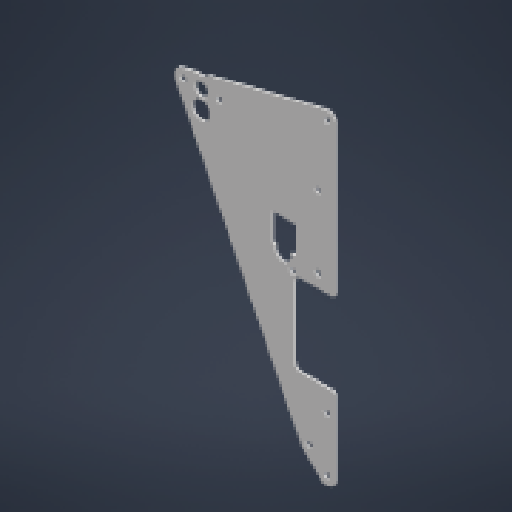
# Autodesk Inventor part: outer-tower-support-proto
Saved by Autodesk Inventor 2023 (Build 270158000, 158)
## iProperties
Created: 2023-03-21
Part Number: outer-tower-support-proto
Material: Generic
Document SubType Name: Modeling
Designer: Liam
Density: 1 g/cm^3
Appearance: Default
Author: Liam
Autodesk Inventor part; units mm, degrees
ref_plane "YZ Plane" through (0, 0, 0) normal (1, 0, 0) x (0, 1, 0)
ref_plane "XZ Plane" through (0, 0, 0) normal (0, 1, 0) x (-1, 0, 0)
ref_plane "XY Plane" through (0, 0, 0) normal (0, 0, 1) x (1, 0, 0)
sketch "Sketch1" plane through (0, 0, 0) normal (0, 0, 1) x (1, 0, 0)
  circle A0 centre (-71.4375, -30.1625) radius 6.35
  line L0 (12.9724, -214.0401) -> (0.2724, -201.3401)
  line L1 (-0.9271, -199.6696) -> (-89.8271, -20.2821)
  line L2 (23.8157, 7.5349) -> (23.8157, -44.8526)
  arc A1 (12.9724, -214.0401) -> (23.8125, -209.55) centre (17.4625, -209.55) ccw
  arc A2 (-0.9271, -199.6696) -> (0.2724, -201.3401) centre (4.7625, -196.85) ccw
  arc A3 (-85.6776, -11.3021) -> (-89.8271, -20.2821) centre (-84.1375, -17.4625) ccw
  arc A4 (23.8157, 7.5349) -> (15.9224, 14.0979) centre (17.4787, 7.9416) ccw
  circle A5 centre (-71.4375, -17.4625) radius 2.1844
  line L3 (-85.6776, -11.3021) -> (-75.211, -8.6854)
  line L4 (15.9224, 14.0979) -> (-66.2619, -6.4482)
  arc A6 (-73.1895, -8.8477) -> (-67.9692, -7.5426) centre (-71.4375, -4.7625) ccw
  arc A7 (-66.2619, -6.4482) -> (-67.9692, -7.5426) centre (-65.4918, -9.5284) ccw
  arc A8 (-73.1895, -8.8477) -> (-75.211, -8.6854) centre (-74.4409, -11.7656) ccw
  circle A9 centre (-71.4375, -17.4625) radius 4.445
  circle A10 centre (11.1125, -88.9) radius 2.2098
  line L5 (23.8125, -159.2779) -> (23.8125, -209.55)
  line L6 (23.8157, -44.8526) -> (23.8157, -94.965)
  circle A11 centre (17.4787, 7.9416) radius 2.1082
  circle A12 centre (-84.1375, -17.4625) radius 2.1082
  circle A13 centre (-58.7375, -17.4625) radius 2.1844 projected
  circle A14 centre (11.1125, -38.1) radius 2.1844 projected
  circle A15 centre (17.4625, -209.55) radius 2.1082
  circle A16 centre (4.7625, -196.85) radius 2.1082
  circle A17 centre (-13.7795, -88.1118) radius 2.0955 projected
  line L7 (-21.3274, -85.3813) -> (-21.3274, -67.4667)
  line L8 (-20.6924, -66.8317) -> (-4.8945, -66.8317)
  line L9 (-4.2595, -67.4667) -> (-4.2595, -85.3813)
  arc A18 (-19.4799, -86.7943) -> (-8.0791, -86.7943) centre (-13.7795, -88.1118) ccw
  line L10 (-7.4604, -86.0163) -> (-4.8945, -86.0163)
  line L11 (-20.0986, -86.0163) -> (-20.6924, -86.0163)
  arc A19 (-7.4604, -86.0163) -> (-8.0791, -86.7943) centre (-7.4604, -86.6513) ccw
  arc A20 (-19.4799, -86.7943) -> (-20.0986, -86.0163) centre (-20.0986, -86.6513) ccw
  arc A21 (-21.3274, -85.3813) -> (-20.6924, -86.0163) centre (-20.6924, -85.3813) ccw
  arc A22 (-4.8945, -86.0163) -> (-4.2595, -85.3813) centre (-4.8945, -85.3813) ccw
  arc A23 (-4.2595, -67.4667) -> (-4.8945, -66.8317) centre (-4.8945, -67.4667) ccw
  arc A24 (-20.6924, -66.8317) -> (-21.3274, -67.4667) centre (-20.6924, -67.4667) ccw
  circle A25 centre (-6.9397, -96.4319) radius 2.1082
  line L12 (-5.5975, -152.05) -> (-5.5975, -101.95)
  line L13 (-1.7875, -155.86) -> (20.6375, -155.86)
  line L14 (23.8125, -159.035) -> (23.8125, -159.2779)
  line L15 (-1.7875, -98.14) -> (20.6407, -98.14)
  arc A26 (-5.5975, -152.05) -> (-1.7875, -155.86) centre (-1.7875, -152.05) ccw
  arc A27 (-1.7875, -98.14) -> (-5.5975, -101.95) centre (-1.7875, -101.95) ccw
  arc A28 (23.8125, -159.035) -> (20.6375, -155.86) centre (20.6375, -159.035) ccw
  arc A29 (20.6407, -98.14) -> (23.8157, -94.965) centre (20.6407, -94.965) ccw
  circle A30 centre (17.4625, -171.45) radius 2.1844 projected
  point P0 (0, 0)
  point P1 (-74.0123, -8.3858)
  point P2 (-67.4605, -6.7478)
  point P3 (16.6133, -60.3277)
  point P4 (-19.242, -86.0163)
  point P5 (-8.317, -86.0163)
  dimension "d13" = 12.7
  dimension "d30" = 4.3688
  dimension "d32" = 3.175
  dimension "d33" = 8.89
  dimension "d34" = 4.4196
  dimension "d51" = 4.2164
  dimension "d52" = 4.2164
  dimension "d54" = 4.2164
  dimension "d55" = 4.2164
  dimension "d56" = 0.635
  dimension "d59" = 4.2164
  dimension "d62" = 3.175
  constraints: 40 point on circle, 32 end point, 27 centre point, 20 tangent, 7 equal radius, 5 coincident, 5 point on line, 4 horizontal, 3 perpendicular, 3 vertical, 1 parallel, 8 other
  measures "d13" diameter of A0
  measures "d30" diameter of A5
  measures "d32" radius of A7
  measures "d33" diameter of A9
  measures "d34" diameter of A10
  measures "d51" diameter of A11
  measures "d52" diameter of A12
  measures "d54" diameter of A15
  measures "d55" diameter of A16
  measures "d56" radius of A19
  measures "d59" diameter of A25
  measures "d62" radius of A28
extrude "Extrusion6" add sketch "Sketch1" along normal blind 1.524 contours L0 A2 L1 A3 L3 A8 A6 A7 L4 A4 L2 L6 A29 L15 A27 L12 A26 L13 A28 L14 L5 A1
body "Solid6"
